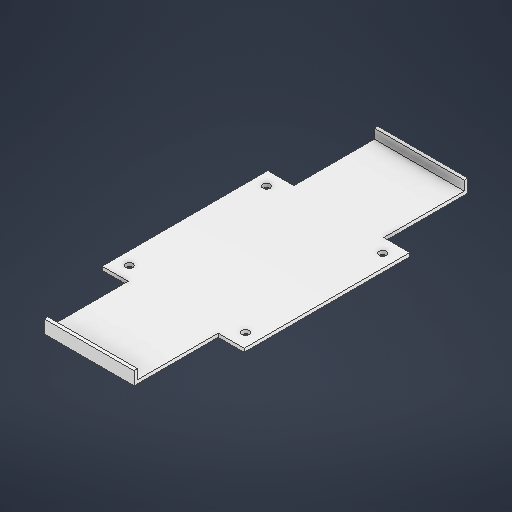
# Autodesk Inventor part: Soporte_bateria_p1
Saved by Autodesk Inventor 2026 (Build 300175050, 175E)
## iProperties
Created: 2025-08-28
Part Number: Soporte_bateria_p1
Material: Plástico ABS
Document SubType Name: Modeling
Designer: rodri
Density: 1.06 g/cm^3
Appearance: Suave - Blanco
Author: rodri
## iProperties of the stored document Soporte_bateria_p1_3DPrint.ipt
Created: 2025-08-28
Part Number: Soporte_bateria_p1_3DPrint
Material: Genérico
Document SubType Name: Modeling
Designer: rodri
Density: 1 g/cm^3
Appearance: Valor por defecto
Author: rodri
Autodesk Inventor part; units mm, degrees
ref_plane "YZ Plane" through (0, 0, 0) normal (1, 0, 0) x (0, 1, 0)
ref_plane "XZ Plane" through (0, 0, 0) normal (0, 1, 0) x (-1, 0, 0)
ref_plane "XY Plane" through (0, 0, 0) normal (0, 0, 1) x (1, 0, 0)
sketch "Boceto1" plane through (0, 0, 0) normal (0, 1, 0) x (-1, 0, 0)
  line L0 (-19, -70.5) -> (19, -70.5)
  line L1 (19, -70.5) -> (19, 70.5)
  line L2 (19, 70.5) -> (-19, 70.5)
  line L3 (-19, 70.5) -> (-19, -70.5)
  line L4 (-19, -70.5) -> (19, 70.5) construction
  line L5 (19, -70.5) -> (-19, 70.5) construction
  line L6 (-30, -35) -> (30, -35)
  line L7 (30, -35) -> (30, 35)
  line L8 (30, 35) -> (-30, 35)
  line L9 (-30, 35) -> (-30, -35)
  line L10 (-30, -35) -> (30, 35) construction
  line L11 (30, -35) -> (-30, 35) construction
  point P0 (0, 0)
  point P1 (-19, 35)
  point P2 (-19, -35)
  point P3 (19, -35)
  point P4 (19, 35)
  dimension "d0" = 141
  dimension "d1" = 38
  dimension "d2" = 70
  dimension "d3" = 60
  constraints: 24 end point, 4 midpoint, 4 parallel, 2 horizontal, 2 perpendicular
  measures "d0" distance of L0.end L1.end
  measures "d1" distance of L1.end L2.end
  measures "d2" distance of L8.end L6.start
  measures "d3" distance of L7.end L8.end
extrude "Extrusión1" add sketch "Boceto1" along normal blind 1.5
sketch "Boceto2" plane through (0, 1.5, 0) normal (0, 1, 0) x (1, 0, 0)
  line L0 (24.55, 29) -> (-24.55, 29)
  line L1 (-24.55, 29) -> (-24.55, -29)
  line L2 (-24.55, -29) -> (24.55, -29)
  line L3 (24.55, -29) -> (24.55, 29)
  line L4 (24.55, 29) -> (-24.55, -29) construction
  line L5 (-24.55, 29) -> (24.55, -29) construction
  point P0 (0, 0)
  dimension "d6" = 49.1
  dimension "d7" = 58
  constraints: 12 end point, 2 midpoint, 2 parallel, 1 horizontal, 1 perpendicular
  measures "d6" distance of L1.end L2.end
  measures "d7" distance of L0.end L1.end
hole "Agujero1" at (-24.55, 1.5, 29) at (-24.55, 1.5, -29) at (24.55, 1.5, -29) at (24.55, 1.5, 29) direction (0, -1, 0) diameter 3.1 end through all clearance for "Tornillo para maquinaria de cabeza plana" size "M2.5" standard "Perfil M métrico ANSI"
sketch "Boceto3" plane through (0, 1.5, 0) normal (0, 1, 0) x (1, 0, 0)
  line L0 (-19, -35) -> (-19, -70.5) projected
  line L1 (19, -70.5) -> (19, -35) projected
  line L2 (-19, -70.5) -> (19, -70.5)
  line L3 (19, -70.5) -> (19, -69)
  line L4 (19, -69) -> (-19, -69)
  line L5 (-19, -69) -> (-19, -70.5)
  point P0 (0, 0)
  point P1 (19, -70.5)
  dimension "d15" = 1.5
  constraints: 8 end point, 2 parallel, 1 horizontal, 1 perpendicular, 1 point on line
  measures "d15" distance between parallel lines of L2 L4
extrude "Extrusión2" add sketch "Boceto3" along normal blind 4
mirror "Simetría1" about plane through (0, 0, 0) normal (0, 0, 1) of "Extrusión2"
